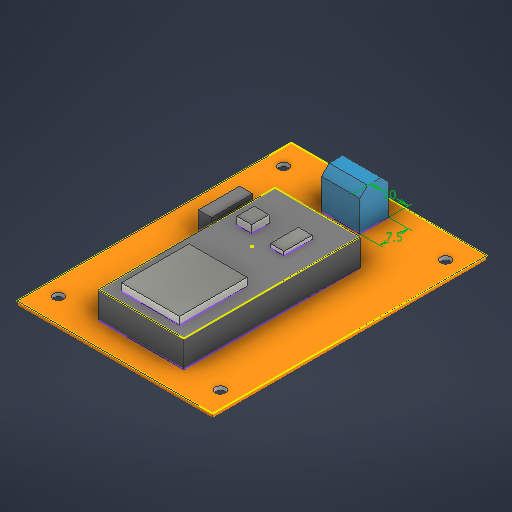
# Autodesk Inventor part: PCB
Saved by Autodesk Inventor 2027.1 (Build 311270010, 270A)
## iProperties
Created: 2026-08-16
Part Number: PCB
Material: Genérico
Document SubType Name: Modeling
Designer: Evellyn
Density: 1 g/cm^3
Appearance: Padrão
Author: Evellyn
Autodesk Inventor part; units mm, degrees
ref_plane "YZ Plane" through (0, 0, 0) normal (1, 0, 0) x (0, 1, 0)
ref_plane "XZ Plane" through (0, 0, 0) normal (0, 1, 0) x (-1, 0, 0)
ref_plane "XY Plane" through (0, 0, 0) normal (0, 0, 1) x (1, 0, 0)
sketch "Esboço1" plane through (0, 0, 0) normal (0, 1, 0) x (-1, 0, 0)
  line L0 (-25.5, 35.75) -> (25.5, 35.75)
  line L1 (25.5, 35.75) -> (25.5, -35.75)
  line L2 (25.5, -35.75) -> (-25.5, -35.75)
  line L3 (-25.5, -35.75) -> (-25.5, 35.75)
  line L4 (-25.5, 35.75) -> (25.5, -35.75) construction
  line L5 (25.5, 35.75) -> (-25.5, -35.75) construction
  circle A0 centre (21.15, 29.4) radius 1.35
  circle A1 centre (-21.15, 29.4) radius 1.35
  line L6 (35.4001, 0) -> (-36.6047, 0)
  circle A2 centre (21.15, -29.4) radius 1.35
  circle A3 centre (-21.15, -29.4) radius 1.35
  point P0 (0, 0)
  dimension "d0" = 51
  dimension "d1" = 71.5
  dimension "d2" = 2.7
  dimension "d3" = 3
  dimension "d4" = 5
  dimension "d5" = 2.7
  dimension "d6" = 5
  dimension "d7" = 3
  dimension "d25" = 6.35
  constraints: 14 end point, 4 centre point, 2 horizontal, 2 midpoint, 2 parallel, 2 symmetric about line, 1 perpendicular, 2 other
  measures "d0" distance of L1.end L2.end
  measures "d1" distance of L0.end L1.end
  measures "d2" diameter of A0
  measures "d3" distance edge to line of A0 L1
  measures "d4" distance edge to line of A0 L0
  measures "d5" diameter of A1
  measures "d6" distance edge to line of A1 L0
  measures "d7" distance edge to line of A1 L3
  measures "d25" distance from line of L2 A2.centre
extrude "Extrusão1" add sketch "Esboço1" along normal blind 1
sketch "Esboço2" plane through (0, 1, 0) normal (0, 1, 0) x (1, 0, 0)
  line L0 (-25.5, 35.75) -> (-25.5, -35.75) projected
  line L1 (-25.5, -35.75) -> (25.5, -35.75) projected
  line L2 (25.5, 35.75) -> (-25.5, 35.75) projected
  line L3 (25.5, -35.75) -> (25.5, 35.75) projected
  line L4 (-10.4597, -29.5298) -> (11.731, -29.5298)
  line L5 (11.731, -29.5298) -> (11.731, 16.4696)
  line L6 (11.731, 16.4696) -> (-10.4597, 16.4696)
  line L7 (-10.4597, 16.4696) -> (-10.4597, -29.5298)
  line L8 (-15.4294, 1.4447) -> (-11.9622, 1.4447)
  line L9 (-11.9622, 1.4447) -> (-11.9622, 12.1933)
  line L10 (-11.9622, 12.1933) -> (-15.4294, 12.1933)
  line L11 (-15.4294, 12.1933) -> (-15.4294, 1.4447)
  line L12 (-5.9522, 24.0977) -> (4.0478, 24.0977)
  line L13 (4.0478, 24.0977) -> (4.0478, 31.5977)
  line L14 (4.0478, 31.5977) -> (-5.9522, 31.5977)
  line L15 (-5.9522, 31.5977) -> (-5.9522, 24.0977)
  point P0 (0, 0)
  dimension "d12" = 10
  dimension "d13" = 7.5
  constraints: 24 end point, 6 parallel, 3 horizontal, 3 perpendicular
  measures "d12" distance of L14.end L13.end
  measures "d13" distance of L13.end L12.end
extrude "Extrusão2" add sketch "Esboço2" along normal blind 7 contours L7 L6 L5 L4 | L11 L10 L9 L8
extrude "Extrusão3" add sketch "Esboço2" along normal blind 10 contours L15 L14 L13 L12
chamfer "Chanfro1" distance 2 angle 45 2 edges at (-0.9522, 11, -24.0977) (-0.9522, 11, -31.5977)
sketch "Esboço3" plane through (0, 8, 0) normal (0, 1, 0) x (1, 0, 0)
  line L0 (-10.4597, 16.4696) -> (-10.4597, -29.5298) projected
  line L1 (-10.4597, -29.5298) -> (11.731, -29.5298) projected
  line L2 (11.731, 16.4696) -> (-10.4597, 16.4696) projected
  line L3 (11.731, -29.5298) -> (11.731, 16.4696) projected
  line L4 (-6.9899, -27.068) -> (8.1586, -27.068)
  line L5 (8.1586, -27.068) -> (8.1586, -9.4197)
  line L6 (8.1586, -9.4197) -> (-6.9899, -9.4197)
  line L7 (-6.9899, -9.4197) -> (-6.9899, -27.068)
  line L8 (-6.9899, 3.0291) -> (-3.1403, 3.0291)
  line L9 (-3.1403, 3.0291) -> (-3.1403, 7.5786)
  line L10 (-3.1403, 7.5786) -> (-6.9899, 7.5786)
  line L11 (-6.9899, 7.5786) -> (-6.9899, 3.0291)
  line L12 (2.5592, 2.2291) -> (6.1088, 2.2291)
  line L13 (6.1088, 2.2291) -> (6.1088, 9.5784)
  line L14 (6.1088, 9.5784) -> (2.5592, 9.5784)
  line L15 (2.5592, 9.5784) -> (2.5592, 2.2291)
  point P0 (0, 0)
  constraints: 24 end point, 6 parallel, 3 horizontal, 3 perpendicular
extrude "Extrusão4" add sketch "Esboço3" along normal blind 2 contours L7 L6 L5 L4 | L11 L10 L9 L8
extrude "Extrusão5" add sketch "Esboço3" along normal blind 1 contours L15 L14 L13 L12
